Aluminium Profiles 20x20 (Autodesk Fusion 360 design; units mm, degrees)
Autodesk Fusion 360 part; units mm, degrees
sketch "Sketch1" plane through (0, 0, 0) normal (0, 1, 0) x (1, 0, 0)
  line L0 (10, 10) -> (-10, 10)
  line L1 (-10, 10) -> (-10, -10)
  line L2 (-10, -10) -> (10, -10)
  line L3 (10, -10) -> (10, 10)
  line L4 (10, 10) -> (-10, -10) construction
  line L5 (-10, 10) -> (10, -10) construction
  line L6 (20, 10) -> (20, -10)
  line L7 (20, -10) -> (40, -10)
  line L8 (40, -10) -> (40, 10)
  line L9 (40, 10) -> (20, 10)
  line L10 (50, 10) -> (50, -10)
  line L11 (50, -10) -> (70, -10)
  line L12 (70, -10) -> (70, 10)
  line L13 (70, 10) -> (50, 10)
  line L14 (100, 10) -> (80, 10)
  line L15 (80, 10) -> (80, -10)
  line L16 (80, -10) -> (100, -10)
  line L17 (100, -10) -> (100, 10)
  dimension "d1" = 20
  dimension "d2" = 20
  dimension "d5" = 20
  dimension "d6" = 20
  dimension "d9" = 20
  dimension "d10" = 20
  dimension "d145" = 20
  dimension "d146" = 20
  constraint perpendicular L0 L1
  constraint parallel L0 L2
  constraint parallel L1 L3
  constraint horizontal L0
  constraint coincident L4 origin
  constraint coincident L5 origin
  constraint perpendicular L6 L9
  constraint parallel L7 L9
  constraint parallel L6 L8
  constraint horizontal L9
  constraint perpendicular L10 L13
  constraint parallel L11 L13
  constraint parallel L10 L12
  constraint horizontal L13
  constraint perpendicular L14 L15
  constraint parallel L14 L16
  constraint parallel L15 L17
  constraint horizontal L14
  measures "d1" distance of L0.end L1.end
  measures "d2" distance of L1.end L2.end
  measures "d5" distance of L6.end L6.start
  measures "d6" distance of L7.end L6.end
  measures "d9" distance of L10.start L10.end
  measures "d10" distance of L11.end L10.end
  measures "d145" distance of L14.end L15.end
  measures "d146" distance of L16.end L15.end
extrude "Extrude1" add sketch "Sketch1" along normal blind 317 contours L0 L1 L2 L3 makes body 1
extrude "Extrude2" add sketch "Sketch1" along normal blind 389 separate body contours L6 L7 L8 L9 makes body 2
extrude "Extrude3" add sketch "Sketch1" along normal blind 82 separate body contours L10 L11 L12 L13 makes body 3
extrude "Extrude4" add sketch "Sketch1" along normal blind 277 separate body contours L14 L15 L16 L17 makes body 4
sketch "Sketch2" plane through (0, 0, 10) normal (0, 0, 1) x (-1, 0, 0)
  line L0 (-80, 0) -> (-100, 0)
  line L1 (-100, 0) -> (-100, -277)
  line L2 (-100, -277) -> (-80, -277)
  line L3 (-80, -277) -> (-80, 0)
  line L4 (-100, -277) -> (-80, 0) construction
  circle A0 centre (-90, -138.5) radius 4.1
  dimension "d149" = 8.2
  constraint coincident L1.end L2.start
  constraint coincident L0.start L3.end
  constraint midpoint L4 A0.centre
  measures "d149" diameter of A0
extrude "Extrude5" cut sketch "Sketch2" against normal through all contours A0 bodies 4
copy_body "Body->Comp1" bodies 3 removing the originals makes body 5 in component "Profile_20x20x82"
copy_body "Body->Comp2" bodies 1 removing the originals makes body 6 in component "Profile_20x20x317"
copy_body "Body->Comp3" bodies 2 removing the originals makes body 7 in component "Profile_20x20x389"
copy_body "Body->Comp4" bodies 4 removing the originals makes body 8 in component "Profile_20x20x277"
sketch "Sketch1 (2)" plane through (0, 0, 0) normal (0, 0, 1) x (1, 0, 0) in component "Corner Structure v3"
  line L0 (0, 0) -> (-45, 0)
  line L1 (0, 0) -> (0, 45)
  line L2 (0, 45) -> (-45, 0)
  line L3 (-5, 40) -> (-5, 5)
  line L4 (-5, 5) -> (-40, 5)
  line L5 (-2, 43) -> (0, 43)
  line L6 (-43, 2) -> (-43, 0)
  dimension "d1_1" = 45
  dimension "d2_1" = 45
  dimension "d5_1" = 5
  dimension "d6_1" = 5
  dimension "d7_1" = 2
  dimension "d8_1" = 2
  constraint coincident L0.start L1.start
  constraint horizontal L0
  constraint perpendicular L0 L1
  constraint coincident L2 L3.start
  constraint parallel L1 L3
  constraint coincident L2 L4.end
  constraint perpendicular L3 L4
  constraint coincident L2 L5.start
  constraint coincident L1 L5.end
  constraint perpendicular L1 L5
  constraint coincident L2 L6.start
  constraint coincident L0 L6.end
  constraint perpendicular L0 L6
  measures "d1_1" distance of L0.start L0.end
  measures "d2_1" distance of L0.start L1.end
  measures "d5_1" vertical distance of L0.start L3.end
  measures "d6_1" horizontal distance of L0.start L3.end
  measures "d7_1" distance of L0.end L6.end
  measures "d8_1" distance of L1.end L5.end
extrude "Extrude2'" add sketch "Sketch1 (2)" along normal blind 20 separate body contours L0 L1 L2 L3 L4 L5 L6 makes body 9 in component "Corner Structure v3"
extrude "Extrude3'" add sketch "Sketch1 (2)" along normal blind 5 contours L2 L3 L4 bodies 9 in component "Corner Structure v3"
sketch "Sketch1 (3)" plane through (0, 0, 0) normal (0, 0, 1) x (1, 0, 0) in component "Corner Structure v3 (1)"
  line L0 (0, 0) -> (-45, 0)
  line L1 (0, 0) -> (0, 45)
  line L2 (0, 45) -> (-45, 0)
  line L3 (-5, 40) -> (-5, 5)
  line L4 (-5, 5) -> (-40, 5)
  line L5 (-2, 43) -> (0, 43)
  line L6 (-43, 2) -> (-43, 0)
  dimension "d1_2" = 45
  dimension "d2_2" = 45
  dimension "d5_2" = 5
  dimension "d6_2" = 5
  dimension "d7_2" = 2
  dimension "d8_2" = 2
  constraint coincident L0.start L1.start
  constraint horizontal L0
  constraint perpendicular L0 L1
  constraint coincident L2 L3.start
  constraint parallel L1 L3
  constraint coincident L2 L4.end
  constraint perpendicular L3 L4
  constraint coincident L2 L5.start
  constraint coincident L1 L5.end
  constraint perpendicular L1 L5
  constraint coincident L2 L6.start
  constraint coincident L0 L6.end
  constraint perpendicular L0 L6
  measures "d1_2" distance of L0.start L0.end
  measures "d2_2" distance of L0.start L1.end
  measures "d5_2" vertical distance of L0.start L3.end
  measures "d6_2" horizontal distance of L0.start L3.end
  measures "d7_2" distance of L0.end L6.end
  measures "d8_2" distance of L1.end L5.end
extrude "Extrude2''" add sketch "Sketch1 (3)" along normal blind 20 separate body contours L0 L1 L2 L3 L4 L5 L6 makes body 10 in component "Corner Structure v3 (1)"
extrude "Extrude3''" add sketch "Sketch1 (3)" along normal blind 5 contours L2 L3 L4 bodies 10 in component "Corner Structure v3 (1)"
sketch "Sketch1 (4)" plane through (0, 0, 0) normal (0, 0, 1) x (1, 0, 0) in component "Corner Structure v3 (2)"
  line L0 (0, 0) -> (-45, 0)
  line L1 (0, 0) -> (0, 45)
  line L2 (0, 45) -> (-45, 0)
  line L3 (-5, 40) -> (-5, 5)
  line L4 (-5, 5) -> (-40, 5)
  line L5 (-2, 43) -> (0, 43)
  line L6 (-43, 2) -> (-43, 0)
  dimension "d1_3" = 45
  dimension "d2_3" = 45
  dimension "d5_3" = 5
  dimension "d6_3" = 5
  dimension "d7_3" = 2
  dimension "d8_3" = 2
  constraint coincident L0.start L1.start
  constraint horizontal L0
  constraint perpendicular L0 L1
  constraint coincident L2 L3.start
  constraint parallel L1 L3
  constraint coincident L2 L4.end
  constraint perpendicular L3 L4
  constraint coincident L2 L5.start
  constraint coincident L1 L5.end
  constraint perpendicular L1 L5
  constraint coincident L2 L6.start
  constraint coincident L0 L6.end
  constraint perpendicular L0 L6
  measures "d1_3" distance of L0.start L0.end
  measures "d2_3" distance of L0.start L1.end
  measures "d5_3" vertical distance of L0.start L3.end
  measures "d6_3" horizontal distance of L0.start L3.end
  measures "d7_3" distance of L0.end L6.end
  measures "d8_3" distance of L1.end L5.end
extrude "Extrude2'''" add sketch "Sketch1 (4)" along normal blind 20 separate body contours L0 L1 L2 L3 L4 L5 L6 makes body 11 in component "Corner Structure v3 (2)"
extrude "Extrude3'''" add sketch "Sketch1 (4)" along normal blind 5 contours L2 L3 L4 bodies 11 in component "Corner Structure v3 (2)"
sketch "Sketch1 (5)" plane through (0, 0, 0) normal (0, 0, 1) x (1, 0, 0) in component "Corner Structure v3 (3)"
  line L0 (0, 0) -> (-45, 0)
  line L1 (0, 0) -> (0, 45)
  line L2 (0, 45) -> (-45, 0)
  line L3 (-5, 40) -> (-5, 5)
  line L4 (-5, 5) -> (-40, 5)
  line L5 (-2, 43) -> (0, 43)
  line L6 (-43, 2) -> (-43, 0)
  dimension "d1_4" = 45
  dimension "d2_4" = 45
  dimension "d5_4" = 5
  dimension "d6_4" = 5
  dimension "d7_4" = 2
  dimension "d8_4" = 2
  constraint coincident L0.start L1.start
  constraint horizontal L0
  constraint perpendicular L0 L1
  constraint coincident L2 L3.start
  constraint parallel L1 L3
  constraint coincident L2 L4.end
  constraint perpendicular L3 L4
  constraint coincident L2 L5.start
  constraint coincident L1 L5.end
  constraint perpendicular L1 L5
  constraint coincident L2 L6.start
  constraint coincident L0 L6.end
  constraint perpendicular L0 L6
  measures "d1_4" distance of L0.start L0.end
  measures "d2_4" distance of L0.start L1.end
  measures "d5_4" vertical distance of L0.start L3.end
  measures "d6_4" horizontal distance of L0.start L3.end
  measures "d7_4" distance of L0.end L6.end
  measures "d8_4" distance of L1.end L5.end
extrude "Extrude2''''" add sketch "Sketch1 (5)" along normal blind 20 separate body contours L0 L1 L2 L3 L4 L5 L6 makes body 12 in component "Corner Structure v3 (3)"
extrude "Extrude3''''" add sketch "Sketch1 (5)" along normal blind 5 contours L2 L3 L4 bodies 12 in component "Corner Structure v3 (3)"
component "Profile_20x20x82" placed x (1, 0, 0) y (0, 0, 1) z (0, -1, 0) at (-88.5214, -13.0886, 13.8372)
component "Profile_20x20x317" placed x (1, 0, 0) y (0, 1, 0) z (0, 0, 1) at (-28.5214, -23.0886, 3.8372)
component "Profile_20x20x389" placed x (0, 1, 0) y (-1, 0, 0) z (0, 0, 1) at (370.4786, -43.0886, 3.8372)
component "Profile_20x20x277" placed x (1, 0, 0) y (0, 1, 0) z (0, 0, 1) at (29.9786, -3.0886, 105.8372)
component "Profile_20x20x317" placed x (-1, 0, 0) y (0, -1, 0) z (0, 0, 1) at (380.4786, 293.9114, 3.8372)
component "Profile_20x20x389" placed x (0, 1, 0) y (-1, 0, 0) z (0, 0, 1) at (370.4786, 253.9114, 3.8372)
component "Profile_20x20x317" placed x (1, 0, 0) y (0, 1, 0) z (0, 0, 1) at (-28.5214, -23.0886, 105.8372)
component "Profile_20x20x389" placed x (0, 1, 0) y (-1, 0, 0) z (0, 0, 1) at (370.4786, -43.0886, 105.8372)
component "Profile_20x20x317" placed x (-1, 0, 0) y (0, -1, 0) z (0, 0, 1) at (380.4786, 293.9114, 105.8372)
component "Profile_20x20x389" placed x (0, 1, 0) y (-1, 0, 0) z (0, 0, 1) at (370.4786, 253.9114, 105.8372)
component "Profile_20x20x82" placed x (1, 0, 0) y (0, 0, 1) z (0, -1, 0) at (320.4786, -13.0886, 13.8372)
component "Profile_20x20x82" placed x (1, 0, 0) y (0, 0, 1) z (0, -1, 0) at (320.4786, 283.9114, 13.8372)
component "Profile_20x20x82" placed x (1, 0, 0) y (0, 0, 1) z (0, -1, 0) at (-88.5214, 283.9114, 13.8372)
component "Corner Structure v3" placed x (0, 1, 0) y (1, 0, 0) z (0, 0, -1) at (-18.5214, 273.9114, 115.8372)
component "Corner Structure v3 (1)" placed x (-1, 0, 0) y (0, 1, 0) z (0, 0, -1) at (-18.5214, -3.0886, 115.8372)
component "Corner Structure v3 (2)" placed x (1, 0, 0) y (0, -1, 0) z (0, 0, -1) at (370.4786, 273.9114, 115.8372)
component "Corner Structure v3 (3)" placed x (0, -1, 0) y (-1, 0, 0) z (0, 0, -1) at (370.4786, -3.0886, 115.8372)
named bodies: "Profil20x20_317", "Profil20x20_389", "Profil20x20_82", "Profil20x20_277"
